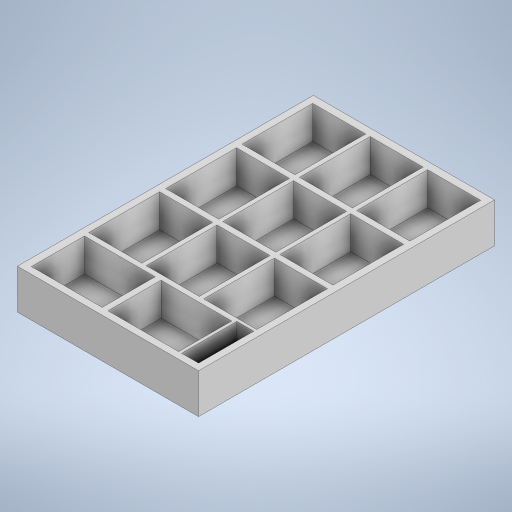
# Autodesk Inventor part: хранитель крпелений
Saved by Autodesk Inventor 2024.2 (Build 282272000, 272)
## iProperties
Created: 2026-01-05
Part Number: хранитель крпелений
Material: Типовые
Document SubType Name: Modeling
Designer: User
Density: 1 g/cm^3
Appearance: По умолчанию
Author: User
Autodesk Inventor part; units mm, degrees
ref_plane "YZ Plane" through (0, 0, 0) normal (1, 0, 0) x (0, 1, 0)
ref_plane "XZ Plane" through (0, 0, 0) normal (0, 1, 0) x (-1, 0, 0)
ref_plane "XY Plane" through (0, 0, 0) normal (0, 0, 1) x (1, 0, 0)
sketch "Эскиз1" plane through (0, 0, 0) normal (0, 1, 0) x (-1, 0, 0)
  line L0 (-41, -75) -> (41, -75)
  line L1 (41, -75) -> (41, 75)
  line L2 (41, 75) -> (-41, 75)
  line L3 (-41, 75) -> (-41, -75)
  line L4 (-41, -75) -> (41, 75) construction
  line L5 (41, -75) -> (-41, 75) construction
  line L6 (41, 75) -> (-41, 75)
  line L7 (-41, 75) -> (-41, 80)
  line L8 (-41, 80) -> (41, 80)
  line L9 (41, 80) -> (41, 75)
  point P0 (0, 0)
  point P1 (-45, 75)
  dimension "d0" = 150
  dimension "d1" = 82
  dimension "d34" = 5
  constraints: 20 end point, 4 parallel, 2 horizontal, 2 midpoint, 2 perpendicular
  measures "d0" distance of L0.end L1.end
  measures "d1" distance of L1.end L2.end
  measures "d34" distance of L8.end L1.end
extrude "Выдавливание1" add sketch "Эскиз1" along normal blind 3
sketch "Эскиз2" plane through (0, 3, 0) normal (0, 1, 0) x (1, 0, 0)
  line L0 (41, 75) -> (-41, 75)
  line L1 (43.9412, 73.2353) -> (-45, -75) construction
  line L2 (-45, 75) -> (45, -75) construction
  line L3 (38, 67.4874) -> (-38, 67.4874)
  line L4 (-38, 67.4874) -> (-38, -67.4874)
  line L5 (38, -67.4874) -> (38, 67.4874)
  line L6 (38, 67.4874) -> (-38, -67.4874) construction
  line L7 (-38, 67.4874) -> (38, -67.4874) construction
  line L8 (40.7632, -80) -> (-41, -80)
  line L9 (-38, -77) -> (-38, -67.4874)
  line L10 (41, -80) -> (41, 75) projected
  line L11 (41, -80) -> (-41, -80)
  line L12 (-41, 75) -> (-41, -80) projected
  line L13 (-41, -80) -> (41, -80)
  line L14 (38, -77) -> (-38, -77)
  line L15 (-41, -77) -> (-41, -80)
  line L16 (-41, -77) -> (-41, 75)
  line L17 (41, -80) -> (41, 75)
  line L18 (38, -67.4874) -> (38, -77)
  point P0 (0, 0)
  dimension "d38" = 3
  dimension "d39" = 3
  constraints: 32 end point, 4 horizontal, 4 point on line, 3 midpoint, 2 parallel, 2 perpendicular, 1 vertical, 6 other
  measures "d39" distance between parallel lines of L8 L14
extrude "Выдавливание2" add sketch "Эскиз2" along normal blind 15
sketch "Эскиз3" plane through (0, 3, 0) normal (0, 1, 0) x (1, 0, 0)
  line L0 (12, -16) -> (-12, -16)
  line L1 (-12, -16) -> (-12, 16)
  line L2 (-12, 16) -> (12, 16)
  line L3 (12, 16) -> (12, -16)
  line L4 (12, -16) -> (-12, 16) construction
  line L5 (-12, -16) -> (12, 16) construction
  line L6 (13, -17.3333) -> (-13, -17.3333)
  line L7 (-13, -17.3333) -> (-13, 17.3333)
  line L8 (-13, 17.3333) -> (13, 17.3333)
  line L9 (13, 17.3333) -> (13, -17.3333)
  line L10 (13, -17.3333) -> (-13, 17.3333) construction
  line L11 (-13, -17.3333) -> (13, 17.3333) construction
  point P0 (0, 0)
  dimension "d8" = 24
  dimension "d9" = 32
  dimension "d10" = 26
  constraints: 24 end point, 4 midpoint, 4 parallel, 2 horizontal, 2 perpendicular, 1 point on line
  measures "d8" distance of L1.end L2.end
  measures "d9" distance of L0.end L1.end
  measures "d10" distance of L7.end L8.end
extrude "Выдавливание3" add sketch "Эскиз3" along normal blind 15
sketch "Эскиз4" plane through (0, 3, 0) normal (0, 1, 0) x (1, 0, 0)
  line L0 (13, 17.3333) -> (-13, 17.3333) projected
  line L1 (-13, 17.3333) -> (-39, 17.3333)
  line L2 (-39, 17.3333) -> (-39, -17.3333)
  line L3 (-39, -17.3333) -> (-13, -17.3333)
  line L4 (-13, -17.3333) -> (-13, 17.3333)
  line L5 (-13.8323, -16) -> (-37.8323, -16)
  line L6 (-37.8323, -16) -> (-37.8323, 16)
  line L7 (-37.8323, 16) -> (-13.8323, 16)
  line L8 (-13.8323, 16) -> (-13.8323, -16)
  line L9 (-13.8323, -16) -> (-37.8323, 16) construction
  line L10 (-37.8323, -16) -> (-13.8323, 16) construction
  line L11 (0, 0) -> (0, 60.0549)
  line L12 (13, 17.3333) -> (39, 17.3333)
  line L13 (39, 17.3333) -> (39, -17.3333)
  line L14 (39, -17.3333) -> (13, -17.3333)
  line L15 (13, -17.3333) -> (13, 17.3333)
  line L16 (13.8323, -16) -> (37.8323, -16)
  line L17 (37.8323, -16) -> (37.8323, 16)
  line L18 (37.8323, 16) -> (13.8323, 16)
  line L19 (13.8323, 16) -> (13.8323, -16)
  line L20 (13.8323, -16) -> (37.8323, 16) construction
  line L21 (37.8323, -16) -> (13.8323, 16) construction
  point P0 (-25.8323, 0)
  point P1 (25.8323, 0)
  dimension "d13" = 26
  dimension "d14" = 24
  dimension "d15" = 32
  constraints: 42 end point, 8 symmetric about line, 4 parallel, 2 horizontal, 2 midpoint, 2 perpendicular, 1 horizontal alignment, 1 vertical
  measures "d13" distance of L0.end L1.end
  measures "d14" distance of L6.end L7.end
  measures "d15" distance of L5.end L6.end
extrude "Выдавливание4" add sketch "Эскиз4" along normal blind 15
sketch "Эскиз6" plane through (0, 3, 0) normal (0, 1, 0) x (1, 0, 0)
  line L0 (38, 17.3333) -> (-38, 17.3333) projected
  line L1 (-39, 17.3333) -> (39, 17.3333)
  line L2 (39, 17.3333) -> (39, 52)
  line L3 (39, 52) -> (-39, 52)
  line L4 (-39, 52) -> (-39, 17.3333)
  line L5 (-39, 17.3333) -> (-13, 17.3333)
  line L6 (-13, 17.3333) -> (-13, 52)
  line L7 (-13, 52) -> (-39, 52)
  line L8 (-39, 52) -> (-39, 17.3333)
  line L9 (-14, 50.6667) -> (-38, 50.6667)
  line L10 (-38, 50.6667) -> (-38, 18.6667)
  line L11 (-38, 18.6667) -> (-14, 18.6667)
  line L12 (-14, 18.6667) -> (-14, 50.6667)
  line L13 (-14, 50.6667) -> (-38, 18.6667) construction
  line L14 (-38, 50.6667) -> (-14, 18.6667) construction
  line L15 (-39, 17.3333) -> (-13, 52)
  line L16 (-39, 52) -> (-13, 17.3333)
  line L17 (0, 0) -> (0, 94.2737)
  line L18 (39, 52) -> (39, 17.3333)
  line L19 (39, 17.3333) -> (13, 17.3333)
  line L20 (13, 17.3333) -> (13, 52)
  line L21 (13, 52) -> (39, 52)
  line L22 (39, 52) -> (39, 17.3333)
  line L23 (14, 50.6667) -> (38, 50.6667)
  line L24 (38, 50.6667) -> (38, 18.6667)
  line L25 (38, 18.6667) -> (14, 18.6667)
  line L26 (14, 18.6667) -> (14, 50.6667)
  line L27 (14, 50.6667) -> (38, 18.6667) construction
  line L28 (38, 50.6667) -> (14, 18.6667) construction
  line L29 (39, 17.3333) -> (13, 52)
  line L30 (39, 52) -> (13, 17.3333)
  line L31 (-13, 17.3333) -> (13, 17.3333)
  line L32 (13, 17.3333) -> (13, 52)
  line L33 (13, 52) -> (-13, 52)
  line L34 (-13, 52) -> (-13, 17.3333)
  line L35 (12, 50.6667) -> (-12, 50.6667)
  line L36 (-12, 50.6667) -> (-12, 18.6667)
  line L37 (-12, 18.6667) -> (12, 18.6667)
  line L38 (12, 18.6667) -> (12, 50.6667)
  line L39 (12, 50.6667) -> (-12, 18.6667) construction
  line L40 (-12, 50.6667) -> (12, 18.6667) construction
  line L41 (0, 0) -> (-32.6399, 0)
  line L42 (39, -17.3333) -> (-39, -17.3333)
  line L43 (-39, -17.3333) -> (39, -17.3333)
  line L44 (39, -17.3333) -> (39, -52)
  line L45 (39, -52) -> (-39, -52)
  line L46 (-39, -52) -> (-39, -17.3333)
  line L47 (-39, -17.3333) -> (-13, -17.3333)
  line L48 (-13, -17.3333) -> (-13, -52)
  line L49 (-13, -52) -> (-39, -52)
  line L50 (-39, -52) -> (-39, -17.3333)
  line L51 (-14, -50.6667) -> (-38, -50.6667)
  line L52 (-38, -50.6667) -> (-38, -18.6667)
  line L53 (-38, -18.6667) -> (-14, -18.6667)
  line L54 (-14, -18.6667) -> (-14, -50.6667)
  line L55 (-14, -50.6667) -> (-38, -18.6667) construction
  line L56 (-38, -50.6667) -> (-14, -18.6667) construction
  line L57 (-39, -17.3333) -> (-13, -52)
  line L58 (-39, -52) -> (-13, -17.3333)
  line L59 (39, -17.3333) -> (13, -17.3333)
  line L60 (38, -18.6667) -> (14, -18.6667)
  line L61 (14, -50.6667) -> (38, -50.6667)
  line L62 (38, -50.6667) -> (38, -18.6667)
  line L63 (14, -18.6667) -> (14, -50.6667)
  line L64 (14, -50.6667) -> (38, -18.6667) construction
  line L65 (38, -50.6667) -> (14, -18.6667) construction
  line L66 (39, -17.3333) -> (13, -52)
  line L67 (39, -52) -> (39, -17.3333)
  line L68 (13, -52) -> (39, -52)
  line L69 (39, -52) -> (39, -17.3333)
  line L70 (39, -52) -> (13, -17.3333)
  line L71 (13, -17.3333) -> (13, -52)
  line L72 (-13, -17.3333) -> (13, -17.3333)
  line L73 (13, -17.3333) -> (13, -52)
  line L74 (13, -52) -> (-13, -52)
  line L75 (-13, -52) -> (-13, -17.3333)
  line L76 (12, -50.6667) -> (-12, -50.6667)
  line L77 (-12, -50.6667) -> (-12, -18.6667)
  line L78 (-12, -18.6667) -> (12, -18.6667)
  line L79 (12, -18.6667) -> (12, -50.6667)
  line L80 (12, -50.6667) -> (-12, -18.6667) construction
  line L81 (-12, -50.6667) -> (12, -18.6667) construction
  point P0 (-26, 34.6667)
  point P1 (26, 34.6667)
  point P2 (0, 34.6667)
  point P3 (-26, -34.6667)
  point P4 (26, -34.6667)
  point P5 (0, -34.6667)
  dimension "d18" = 34.6667
  dimension "d19" = 26
  dimension "d20" = 24
  dimension "d21" = 32
  dimension "d22" = 24
  constraints: 162 end point, 38 symmetric about line, 10 parallel, 6 horizontal, 5 midpoint, 5 perpendicular, 3 point on line, 1 vertical
  measures "d18" distance of L3.end L1.start
  measures "d19" distance of L1.start L5.end
  measures "d20" distance of L10.end L11.end
  measures "d21" distance of L9.end L10.end
  measures "d22" distance of L36.end L37.end
extrude "Выдавливание5" add sketch "Эскиз6" along normal blind 15 contours L0 L30 L25 L29 L1 | L0 L17 L37 L38 L35 L3 L20 | L20 L29 L26 L30 | L29 L24 L30 L2 | L0 L6 L3 L17 L35 L36 L37 | L3 L30 L23 L29 | L16 L12 L15 L6 | L0 L1 L15 L11 L16 | L15 L9 L16 L3 | L4 L16 L10 L15 | L66 L60 L70 L42 | L44 L70 L62 L66 | L71 L45 L48 L42 | L70 L63 L66 L71 | L45 L66 L61 L70 | L58 L53 L57 L42 | L48 L57 L54 L58 | L57 L52 L58 L46 | L45 L58 L51 L57
sketch "Эскиз7" plane through (0, 3, 0) normal (0, 1, 0) x (1, 0, 0)
  line L0 (-37.6667, -53) -> (-5.6667, -53)
  line L1 (-5.6667, -53) -> (-5.6667, -77)
  line L2 (-5.6667, -77) -> (-37.6667, -77)
  line L3 (-37.6667, -77) -> (-37.6667, -53)
  line L4 (-4.3333, -52) -> (-39, -52)
  line L5 (-39, -52) -> (-39, -78)
  line L6 (-39, -78) -> (-4.3333, -78)
  line L7 (-4.3333, -78) -> (-4.3333, -52)
  line L8 (-4.3333, -52) -> (-39, -78) construction
  line L9 (-39, -52) -> (-4.3333, -78) construction
  line L10 (-37.6667, -77) -> (-5.6667, -53)
  line L11 (-5.6667, -77) -> (-37.6667, -53)
  line L12 (-4.3333, -52) -> (30.3333, -52)
  line L13 (30.3333, -52) -> (30.3333, -78)
  line L14 (30.3333, -78) -> (-4.3333, -78)
  line L15 (-4.3333, -78) -> (-4.3333, -52)
  line L16 (29, -53) -> (-3, -53)
  line L17 (-3, -53) -> (-3, -77)
  line L18 (-3, -77) -> (29, -77)
  line L19 (29, -77) -> (29, -53)
  line L20 (29, -53) -> (-3, -77) construction
  line L21 (-3, -53) -> (29, -77) construction
  line L22 (-4.3333, -78) -> (30.3333, -52)
  line L23 (30.3333, -78) -> (-4.3333, -52)
  point P0 (0, 0)
  point P1 (-21.6667, -65)
  point P2 (13, -65)
  dimension "d25" = 24
  dimension "d26" = 32
  dimension "d27" = 26
  dimension "d29" = 34.6667
  dimension "d30" = 34.6667
  dimension "d31" = 32
  constraints: 48 end point, 8 parallel, 6 midpoint, 4 horizontal, 4 perpendicular, 1 coincident, 1 collinear
  measures "d25" distance of L2.end L0.start
  measures "d26" distance of L1.end L2.end
  measures "d27" distance of L4.end L5.end
  measures "d29" distance of L5.end L6.end
  measures "d30" distance of L13.end L14.end
  measures "d31" distance of L17.end L18.end
extrude "Выдавливание6" add sketch "Эскиз7" along normal blind 15 contours L7 L6 L5 L4 | L23 L17 L22 L7 | L12 L22 L16 L23 | L22 L18 L23 L14 | L13 L23 L19 L22
sketch "Эскиз8" plane through (0, 18, 0) normal (0, 1, 0) x (1, 0, 0)
  line L0 (-41, 75) -> (-41, -80) projected
  line L1 (-41, 75) -> (41.8498, 75)
  line L2 (41.8498, 75) -> (41.8498, 52)
  line L3 (41.8498, 52) -> (-41, 52)
  line L4 (-41, 52) -> (-41, 75)
  point P0 (0, 0)
  dimension "d40" = 23
  constraints: 8 end point, 2 parallel, 1 horizontal, 1 perpendicular
  measures "d40" distance of L1.end L2.end
extrude "Выдавливание7" cut sketch "Эскиз8" against normal blind 500
sketch "Эскиз9" plane through (0, 18, 0) normal (0, 1, 0) x (1, 0, 0)
  line L0 (-41, 52) -> (-41, -80) projected
  line L1 (-41, 52) -> (41, 52)
  line L2 (41, 52) -> (41, 54)
  line L3 (41, 54) -> (-41, 54)
  line L4 (-41, 54) -> (-41, 52)
  point P0 (0, 0)
  dimension "d43" = 2
  constraints: 8 end point, 2 parallel, 1 horizontal, 1 perpendicular
  measures "d43" distance of L3.end L0.start
extrude "Выдавливание8" add sketch "Эскиз9" against normal up to surface (18 mm away)
